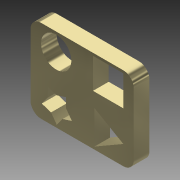
# Autodesk Inventor part: Passener Base
Saved by Autodesk Inventor 2015 (Build 190159000, 159)
## iProperties
Created: 2015-01-16
Part Number: Passener Base
Material: Generic
Document SubType Name: Modeling
Designer: PLTW-Stu-02
Density: 1 g/cm^3
Appearance: Gold - Metal
Author: PLTW-Stu-02
Autodesk Inventor part; units mm, degrees
ref_plane "YZ Plane" through (0, 0, 0) normal (1, 0, 0) x (0, 1, 0)
ref_plane "XZ Plane" through (0, 0, 0) normal (0, 1, 0) x (-1, 0, 0)
ref_plane "XY Plane" through (0, 0, 0) normal (0, 0, 1) x (1, 0, 0)
sketch "Sketch1" plane through (0, 0, 0) normal (0, 0, 1) x (1, 0, 0)
  line L0 (26.7329, 44.7833) -> (66.7379, 44.7833)
  line L1 (71.8179, 39.7033) -> (71.8179, 9.4773)
  line L2 (66.7379, 4.3973) -> (26.7329, 4.3973)
  line L3 (21.6529, 9.4773) -> (21.6529, 39.7033)
  arc A0 (26.7329, 44.7833) -> (21.6529, 39.7033) centre (26.7329, 39.7033) ccw
  arc A1 (21.6529, 9.4773) -> (26.7329, 4.3973) centre (26.7329, 9.4773) ccw
  arc A2 (66.7379, 4.3973) -> (71.8179, 9.4773) centre (66.7379, 9.4773) ccw
  arc A3 (71.8179, 39.7033) -> (66.7379, 44.7833) centre (66.7379, 39.7033) ccw
  circle A4 centre (34.0989, 36.1473) radius 7.366
  line L4 (52.0059, 43.5133) -> (66.7379, 43.5133)
  line L5 (66.7379, 43.5133) -> (66.7379, 28.7813)
  line L6 (66.7379, 28.7813) -> (52.0059, 28.7813)
  line L7 (52.0059, 28.7813) -> (52.0059, 43.5133)
  line L8 (52.7038, 21.8725) -> (66.7379, 13.7699)
  line L9 (66.7379, 13.7699) -> (52.7038, 5.6673)
  line L10 (52.7038, 5.6673) -> (52.7038, 21.8725)
  line L11 (29.9001, 19.5668) -> (34.4164, 18.0994)
  line L12 (34.4164, 18.0994) -> (38.9326, 19.5668)
  line L13 (38.9326, 19.5668) -> (38.9326, 14.8182)
  line L14 (38.9326, 14.8182) -> (41.7238, 10.9764)
  line L15 (41.7238, 10.9764) -> (37.2076, 9.509)
  line L16 (37.2076, 9.509) -> (34.4164, 5.6673)
  line L17 (34.4164, 5.6673) -> (31.6252, 9.509)
  line L18 (31.6252, 9.509) -> (27.1089, 10.9764)
  line L19 (27.1089, 10.9764) -> (29.9001, 14.8182)
  line L20 (29.9001, 14.8182) -> (29.9001, 19.5668)
  point P0 (0, 0)
  point P1 (71.8179, 4.3973)
  point P2 (71.8179, 44.7833)
  point P3 (34.4164, 13.3508)
  dimension "d1" = 40.386
  dimension "d2" = 5.08
  dimension "d3" = 14.732
  dimension "d4" = 12.446
  dimension "d5" = 8.636
  dimension "d6" = 14.732
  dimension "d7" = 14.732
  dimension "d8" = 1.27
  dimension "d9" = 5.08
  dimension "d18" = 16.2052
  constraints: 42 end point, 8 point on circle, 8 tangent, 5 centre point, 4 parallel, 4 point on line, 3 equal radius, 2 horizontal, 2 perpendicular, 2 vertical, 6 other
  measures "d1" distance of point (71.818, 44.783) point (71.818, 4.397)
  measures "d2" radius of A0
  measures "d3" diameter of A4
  measures "d4" horizontal distance of A4.centre L3.end
  measures "d5" vertical distance of A4.centre L0.start
  measures "d6" distance of L5.end L6.end
  measures "d7" distance of L4.end L5.end
  measures "d8" distance between parallel lines of L0 L4
  measures "d9" distance between parallel lines of L1 L5
  measures "d18" distance of L9.end L8.start
extrude "Extrusion2" add sketch "Sketch1" along normal blind 7.62
shell "Shell4" thickness 0.254 removed faces 1 at (62.0598, 21.4745, 0)
body "Solid2"
